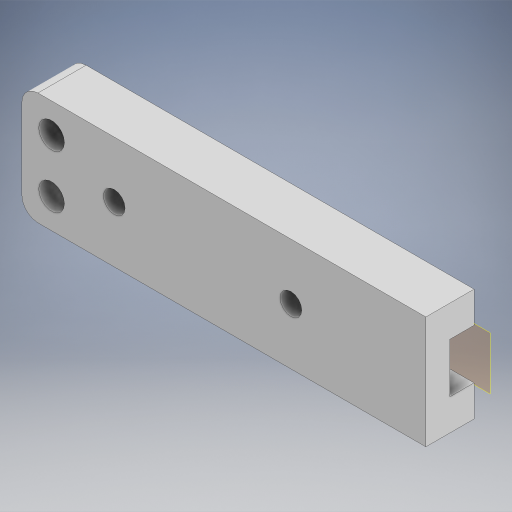
# Autodesk Inventor part: connecting plate under body_zig10
Saved by Autodesk Inventor 2024 (Build 280153000, 153)
## iProperties
Created: 2024-09-11
Part Number: connecting plate under body_zig10
Material: 일반
Document SubType Name: Modeling
Designer: ASUS
Density: 1 g/cm^3
Appearance: 기본값
Author: ASUS
Autodesk Inventor part; units mm, degrees
ref_plane "YZ Plane" through (0, 0, 0) normal (1, 0, 0) x (0, 1, 0)
ref_plane "XZ Plane" through (0, 0, 0) normal (0, 1, 0) x (-1, 0, 0)
ref_plane "XY Plane" through (0, 0, 0) normal (0, 0, 1) x (1, 0, 0)
ref_plane "작업 평면1" through (0, 0, 0) normal (0, 0, 1) x (1, 0, 0)
sketch "스케치1" plane through (0, 0, 0) normal (0, 0, 1) x (1, 0, 0)
  line L0 (-7, 6) -> (-7, 0) projected
  line L1 (-7, 6) -> (-53, 6) projected
  line L2 (-53, 0) -> (-53, 6) projected
  line L3 (-7, 0) -> (-53, 0) projected
  circle A0 centre (-45.5, 2.8) radius 1.35 projected
  circle A1 centre (-23.5, 2.8) radius 1.35 projected
  line L4 (-53.3, -0.3) -> (-53.3, 6.3)
  line L5 (-53.3, 6.3) -> (-6.7, 6.3)
  line L6 (-6.7, 6.3) -> (-6.7, -0.3)
  line L7 (-6.7, -0.3) -> (-53.3, -0.3)
  line L8 (-57, -4) -> (-57, 10)
  line L9 (-57, 10) -> (-3, 10)
  line L10 (-3, 10) -> (-3, -4)
  line L11 (-3, -4) -> (-57, -4)
  line L12 (-6.7, -0.3) -> (-57, -0.3)
  line L13 (-57, -0.3) -> (-57, -4)
  line L14 (-57, -4) -> (-6.7, -4)
  line L15 (-6.7, -4) -> (-6.7, -0.3)
  line L16 (-6.7, 6.3) -> (-57, 6.3)
  line L17 (-57, 6.3) -> (-57, 10)
  line L18 (-57, 10) -> (-6.7, 10)
  line L19 (-6.7, 10) -> (-6.7, 6.3)
  point P0 (0, 0)
  dimension "d0" = 0.3
  dimension "d1" = 4
  constraints: 32 end point, 4 parallel, 2 horizontal, 2 perpendicular, 6 other
  measures "d0" distance between parallel lines of L3 L7
  measures "d1" distance between parallel lines of L3 L11
extrude "돌출1" add sketch "스케치1" along normal blind 3 contours L12 L8 L16 L4 | L7 L15 L11 L8 L12 | L16 L8 L9 L19 L5
sketch "스케치2" plane through (0, 0, 3) normal (0, 0, 1) x (1, 0, 0)
  line L0 (-6.7, -0.3) -> (-53.3, -0.3) projected
  line L1 (-53.3, -0.3) -> (-53.3, 6.3) projected
  line L2 (-53.3, 6.3) -> (-6.7, 6.3) projected
  line L3 (-6.7, 6.3) -> (-6.7, 10) projected
  line L4 (-6.7, 10) -> (-57, 10) projected
  line L5 (-57, 10) -> (-57, -4) projected
  line L6 (-57, -4) -> (-6.7, -4) projected
  line L7 (-6.7, -4) -> (-6.7, -0.3) projected
  line L8 (-6.7, -4) -> (-57, -4)
  line L9 (-57, -4) -> (-57, 10)
  line L10 (-57, 10) -> (-6.7, 10)
  line L11 (-6.7, 10) -> (-6.7, -4)
  line L12 (-7, 6) -> (-7, 0) projected
  line L13 (-7, 6) -> (-53, 6) projected
  line L14 (-53, 0) -> (-53, 6) projected
  line L15 (-7, 0) -> (-53, 0) projected
  circle A0 centre (-45.5, 2.8) radius 1.35 projected
  circle A1 centre (-23.5, 2.8) radius 1.35 projected
  point P0 (0, 0)
  constraints: 8 end point, 2 parallel, 1 horizontal, 1 perpendicular
extrude "돌출2" add sketch "스케치2" along normal blind 3 contours L7 L6 L5 L4 L3 L2 L1 L0 | L0 L1 L2 L11 | L12 L15 L14 L13
sketch "스케치3" plane through (0, 0, 0) normal (0, 0, -1) x (-1, 0, 0)
  line L0 (6.7, -0.3) -> (53.3, -0.3) projected
  line L1 (6.7, -4) -> (6.7, -0.3) projected
  line L2 (57, -4) -> (6.7, -4) projected
  line L3 (57, 10) -> (57, -4) projected
  line L4 (6.7, 10) -> (57, 10) projected
  line L5 (6.7, 6.3) -> (6.7, 10) projected
  line L6 (53.3, 6.3) -> (6.7, 6.3) projected
  line L7 (53.3, -0.3) -> (53.3, 6.3) projected
  point P0 (0, 0)
hole "구멍1" at (-53.3, -0.3, 0) at (-53.3, 6.3, 0) direction (0, 0, 1) diameter 3.2 end through all
fillet "모깎기1" radius 2 2 edges at (-57, -4, 3) (-57, 10, 3)
move faces "이동1" translate (0, 0.2, 0) faces at (-45.23, 4.1227, 5) (-22.1544, 2.6914, 5)
sketch "스케치4" plane through (0, 0, 3) normal (0, 0, -1) x (-1, 0, 0)
  arc A0 (57, 8) -> (55, 10) centre (55, 8) ccw projected
  line L0 (6.7, 10) -> (55, 10) projected
  line L1 (6.7, 6.3) -> (6.7, 10) projected
  line L2 (51.7, 6.3) -> (6.7, 6.3) projected
  arc A1 (53.3, 4.7) -> (51.7, 6.3) centre (53.3, 6.3) ccw projected
  line L3 (53.3, 1.3) -> (53.3, 4.7) projected
  arc A2 (51.7, -0.3) -> (53.3, 1.3) centre (53.3, -0.3) ccw projected
  line L4 (6.7, -0.3) -> (51.7, -0.3) projected
  line L5 (6.7, -4) -> (6.7, -0.3) projected
  line L6 (55, -4) -> (6.7, -4) projected
  arc A3 (55, -4) -> (57, -2) centre (55, -2) ccw projected
  line L7 (57, 8) -> (57, -2) projected
  line L8 (6.7, -0.3) -> (6.7, 6.3) projected
  line L9 (6.7, 6.3) -> (53.3, 6.3)
  line L10 (53.3, 6.3) -> (53.3, -0.3)
  line L11 (53.3, -0.3) -> (6.7, -0.3)
  line L12 (6.7, -0.3) -> (6.7, 6.3)
  line L13 (53.1, 6.1) -> (6.9, 6.1)
  line L14 (6.9, 6.1) -> (6.9, -0.1)
  line L15 (6.9, -0.1) -> (53.1, -0.1)
  line L16 (53.1, -0.1) -> (53.1, 6.1)
  line L17 (53.3, 6.3) -> (53.1, 6.3)
  line L18 (53.1, 6.3) -> (53.1, -0.3)
  line L19 (53.1, -0.3) -> (53.3, -0.3)
  line L20 (53.3, -0.3) -> (53.3, 6.3)
  arc A4 (51.7, 6.3) -> (53.3, 4.7) centre (53.3, 6.3) ccw projected
  line L21 (51.7, 6.3) -> (6.7, 6.3) projected
  line L22 (6.7, -0.3) -> (6.7, 6.3) projected
  line L23 (6.7, -0.3) -> (51.7, -0.3) projected
  arc A5 (53.3, 1.3) -> (51.7, -0.3) centre (53.3, -0.3) ccw projected
  line L24 (53.3, 1.3) -> (53.3, 4.7) projected
  circle A6 centre (23.5, 3) radius 1.35 projected
  circle A7 centre (45.5, 3) radius 1.35 projected
  line L25 (6.9, 6.1) -> (6.7, 6.1)
  line L26 (6.7, 6.1) -> (6.7, -0.1)
  line L27 (6.7, -0.1) -> (6.9, -0.1)
  line L28 (6.9, -0.1) -> (6.9, 6.1)
  point P0 (0, 0)
  point P1 (6.9, -0.1)
  point P2 (6.7, -0.1)
  point P3 (51.7125, -0.1)
  point P4 (51.7125, 6.1)
  dimension "d17" = 0.2
  constraints: 32 end point, 8 parallel, 4 perpendicular, 3 horizontal, 2 point on line, 3 other
  measures "d17" distance between parallel lines of L9 L13
extrude "돌출3" add sketch "스케치4" along normal up to surface (3 mm away) contours L2 A4 L13 L25 L8 | L8 L27 L15 A5 L4
